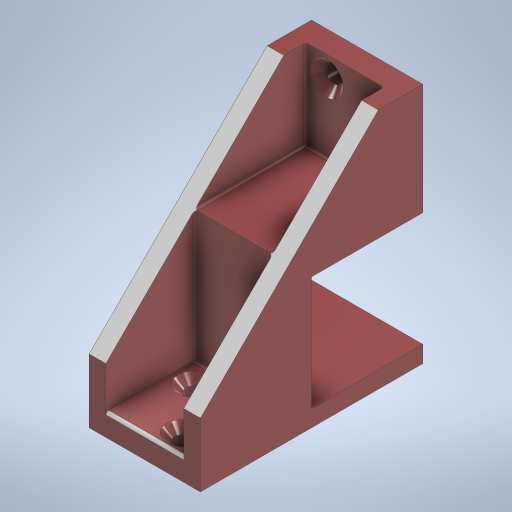
# Autodesk Inventor part: Uniont
Saved by Autodesk Inventor 2024 (Build 280153000, 153)
## iProperties
Created: 2023-07-08
Part Number: Uniont
Material: Genérico
Document SubType Name: Modeling
Designer: sergi
Density: 1 g/cm^3
Appearance: Valor por defecto
Author: sergi
Autodesk Inventor part; units mm, degrees
ref_plane "YZ Plane" through (0, 0, 0) normal (1, 0, 0) x (0, 1, 0)
ref_plane "XZ Plane" through (0, 0, 0) normal (0, 1, 0) x (-1, 0, 0)
ref_plane "Plano de trabajo1" through (0, 0, 0) normal (0, 0, 1) x (1, 0, 0)
sketch "Boceto1" plane through (0, 0, 0) normal (0, 0, 1) x (1, 0, 0)
  line L0 (-395, -200.5) -> (-395, -220.5) projected
  line L1 (-395, -220.5) -> (335, -220.5) projected
  line L2 (335, -200.5) -> (335, -220.5) projected
  line L3 (-395, -200.5) -> (335, -200.5) projected
  line L4 (-145, 767.5) -> (-145, -767.5) projected
  line L5 (-145, -767.5) -> (145, -767.5) projected
  line L6 (145, -767.5) -> (145, 767.5) projected
  line L7 (145, 767.5) -> (-145, 767.5) projected
  line L8 (335.5, -200) -> (335.5, -221)
  line L9 (335.5, -221) -> (-395.5, -221)
  line L10 (-395.5, -221) -> (-395.5, -200)
  line L11 (-395.5, -200) -> (335.5, -200)
  line L12 (-145, -200) -> (-145, -180)
  line L13 (-145, -180) -> (-125, -180)
  line L14 (-125, -180) -> (-125, -200)
  line L15 (-125, -200) -> (-145, -200)
  line L16 (-145, -200) -> (-145, -180)
  point P0 (0, 0)
  dimension "d0" = 0.5
  dimension "d1" = 20
  dimension "d2" = 20
  dimension "d3" = 20
  constraints: 18 end point, 3 point on line, 2 parallel, 1 horizontal, 1 perpendicular, 3 other
  measures "d0" distance between parallel lines of L3 L11
  measures "d1" distance of L12.start L12.end
  measures "d2" distance of L14.end L15.end
  measures "d3" distance of L13.end L14.end
extrude "Extrusión1" add sketch "Boceto1" along normal blind 4 contours L4 L13 L14 L11
sketch "Boceto3" plane through (0, 0, 4) normal (0, 0, 1) x (1, 0, 0)
  line L0 (-125, -180) -> (-145, -180) projected
  line L1 (-145, -180) -> (-145, -200) projected
  line L2 (-145, -200) -> (-125, -200) projected
  line L3 (-125, -200) -> (-125, -180) projected
  line L4 (-145, -200) -> (-125, -200)
  line L5 (-125, -200) -> (-125, -196)
  line L6 (-125, -196) -> (-145, -196)
  line L7 (-145, -196) -> (-145, -200)
  point P0 (0, 0)
  dimension "d6" = 4
  constraints: 8 end point, 2 parallel, 1 horizontal, 1 perpendicular, 1 point on line
  measures "d6" distance of L5.end L4.end
extrude "Extrusión2" add sketch "Boceto3" along normal blind 20 contours L3 L2 L1 L6
sketch "Boceto4" plane through (-145, -200, 0) normal (0, -1, 0) x (1, 0, 0)
  line L0 (0, 0) -> (20, 0) projected
  line L1 (20, 0) -> (20, 24) projected
  line L2 (0, 24) -> (20, 24) projected
  line L3 (0, 0) -> (0, 24) projected
  line L4 (0, 24) -> (20, 24) projected
  line L5 (20, 24) -> (0, 24)
  line L6 (0, 24) -> (0, 20)
  line L7 (0, 20) -> (20, 20)
  line L8 (20, 20) -> (20, 24)
  point P0 (145, 0)
  dimension "d9" = 4
  constraints: 8 end point, 2 parallel, 1 horizontal, 1 perpendicular, 1 point on line
  measures "d9" distance of L6.end L5.end
extrude "Extrusión3" add sketch "Boceto4" along normal blind 20.5 contours L3 L2 L1 L7
sketch "Boceto6" plane through (0, 0, 4) normal (0, 0, 1) x (1, 0, 0)
  line L0 (-145, -196) -> (-125, -196) projected
  line L1 (-125, -196) -> (-125, -180) projected
  line L2 (-125, -180) -> (-145, -180) projected
  line L3 (-145, -180) -> (-145, -196) projected
  line L4 (-145, -180) -> (-142, -180)
  line L5 (-142, -180) -> (-142, -196)
  line L6 (-142, -196) -> (-145, -196)
  line L7 (-145, -196) -> (-145, -180)
  line L8 (-125, -196) -> (-128, -196)
  line L9 (-128, -196) -> (-128, -180)
  line L10 (-128, -180) -> (-125, -180)
  line L11 (-125, -180) -> (-125, -196)
  point P0 (0, 0)
  dimension "d12" = 3
  dimension "d13" = 16
  dimension "d14" = 3
  constraints: 16 end point, 4 parallel, 2 horizontal, 2 perpendicular, 1 point on line
  measures "d12" distance of L5.end L6.end
  measures "d13" distance of L4.end L5.end
  measures "d14" distance of L9.end L10.end
extrude "Extrusión4" add sketch "Boceto6" along normal blind 20 contours L3 L2 L5 L0 | L9 L2 L1 L0
chamfer "Chaflán1" [suppressed]
sketch "Boceto7" plane through (0, 0, 4) normal (0, 0, 1) x (1, 0, 0)
  line L0 (-142, -180) -> (-142, -196) projected
  line L1 (-142, -196) -> (-128, -196) projected
  line L2 (-128, -196) -> (-128, -180) projected
  line L3 (-128, -180) -> (-142, -180) projected
  line L4 (-138.3, -192.3) -> (-138.3, -183.7)
  line L5 (-138.3, -183.7) -> (-131.7, -183.7)
  line L6 (-131.7, -183.7) -> (-131.7, -192.3)
  line L7 (-131.7, -192.3) -> (-138.3, -192.3)
  circle A0 centre (-138.3, -183.7) radius 3
  circle A1 centre (-131.7, -192.3) radius 3
  circle A2 centre (-138.3, -183.7) radius 1.65
  circle A3 centre (-131.7, -192.3) radius 1.65
  point P0 (0, 0)
  dimension "d20" = 3.7
  dimension "d21" = 6
  dimension "d22" = 6
  dimension "d23" = 3.3
  dimension "d24" = 3.3
  constraints: 8 end point, 4 centre point, 4 coincident, 3 other
  measures "d20" distance between parallel lines of L0 L4
  measures "d21" diameter of A0
  measures "d22" diameter of A1
  measures "d23" diameter of A2
  measures "d24" diameter of A3
hole "Agujero1" at (-138.3, -183.7, 4) at (-131.7, -192.3, 4) direction (0, 0, -1) diameter 3.2 end through all countersink diameter 6 countersink angle 90
sketch "Boceto8" plane through (-145, -220.5, 0) normal (0, -1, 0) x (1, 0, 0)
  line L0 (17, 24) -> (17, 4) projected
  line L1 (20, 20) -> (0, 20) projected
  line L2 (0, 0) -> (0, 20) projected
  line L3 (0, 0) -> (20, 0) projected
  line L4 (20, 0) -> (20, 20) projected
  line L5 (20, 20) -> (20, 24) projected
  line L6 (20, 24) -> (0, 24) projected
  line L7 (0, 24) -> (0, 20) projected
  line L8 (0, 20) -> (20, 20) projected
  point P0 (145, 0)
extrude "Extrusión5" add sketch "Boceto8" along normal blind 3
sketch "Boceto9" plane through (0, 0, 24) normal (0, 0, 1) x (1, 0, 0)
  line L0 (-145, -180) -> (-145, -223.5) projected
  line L1 (-125, -223.5) -> (-145, -223.5) projected
  line L2 (-125, -180) -> (-125, -223.5) projected
  line L3 (-128, -196) -> (-142, -196) projected
  line L4 (-145, -223.5) -> (-125, -223.5)
  line L5 (-125, -223.5) -> (-125, -219.5)
  line L6 (-125, -219.5) -> (-145, -219.5)
  line L7 (-145, -219.5) -> (-145, -223.5)
  line L8 (-125, -180) -> (-128, -180) projected
  line L9 (-128, -180) -> (-128, -196) projected
  line L10 (-142, -196) -> (-142, -180) projected
  line L11 (-142, -180) -> (-145, -180) projected
  point P0 (0, 0)
  dimension "d35" = 4
  constraints: 8 end point, 2 parallel, 1 horizontal, 1 perpendicular, 1 point on line
  measures "d35" distance of L5.end L4.end
extrude "Extrusión6" add sketch "Boceto9" along normal blind 16 contours L6 L2 L1 L0
sketch "Boceto10" plane through (-145, -219.5, 24) normal (0, 1, 0) x (1, 0, 0)
  line L0 (0, 0) -> (20, 0) projected
  line L1 (0, 0) -> (0, -16) projected
  line L2 (20, -16) -> (0, -16) projected
  line L3 (20, 0) -> (20, -16) projected
  line L4 (20, -16) -> (17, -16)
  line L5 (17, -16) -> (17, 0)
  line L6 (17, 0) -> (20, 0)
  line L7 (20, 0) -> (20, -16)
  line L8 (0, -16) -> (3, -16)
  line L9 (3, -16) -> (3, 0)
  line L10 (3, 0) -> (0, 0)
  line L11 (0, 0) -> (0, -16)
  point P0 (145, 24)
  point P1 (3, -16)
  point P2 (3, 0)
  point P3 (17, -16)
  dimension "d38" = 3
  dimension "d39" = 3
  dimension "d40" = 16
  constraints: 16 end point, 4 parallel, 2 horizontal, 2 perpendicular, 1 point on line
  measures "d38" distance of L5.end L6.end
  measures "d39" distance of L10.end L9.end
  measures "d40" distance of L9.end L8.end
extrude "Extrusión7" add sketch "Boceto10" along normal up to surface (39.5 mm away) contours L0 L9 L2 L1 | L0 L3 L2 L5
chamfer "Chaflán2" [suppressed]
chamfer "Chaflán3" [suppressed]
sketch "Boceto11" plane through (-142, -219.5, 24) normal (0, 1, 0) x (1, 0, 0)
  line L0 (0, 0) -> (0, -16) projected
  line L1 (14, -16) -> (0, -16) projected
  line L2 (14, -16) -> (14, 0) projected
  line L3 (0, 0) -> (14, 0) projected
  line L4 (3.7, -12.3) -> (3.7, -3.7)
  line L5 (3.7, -3.7) -> (10.3, -3.7)
  line L6 (10.3, -3.7) -> (10.3, -12.3)
  line L7 (10.3, -12.3) -> (3.7, -12.3)
  circle A0 centre (3.7, -3.7) radius 1.6
  circle A1 centre (10.3, -12.3) radius 1.6
  point P0 (142, 24)
  dimension "d49" = 3.7
  dimension "d50" = 3.2
  dimension "d51" = 3.2
  constraints: 8 end point, 2 centre point, 2 coincident, 3 other
  measures "d49" distance between parallel lines of L1 L7
  measures "d50" diameter of A0
  measures "d51" diameter of A1
hole "Agujero2" at (-131.7, -219.5, 36.3) at (-138.3, -219.5, 27.7) direction (0, -1, 0) diameter 3.2 end through all countersink diameter 6 countersink angle 90
fillet "Empalme2" radius 0.5 9 edges at (-135, -219.5, 40) (-142, -207.75, 24) (-128, -207.75, 24) (-135, -219.5, 24) (-142, -196, 14) (-135, -196, 4) (-142, -188, 4) (-128, -188, 4) (-128, -196, 14)
chamfer "Chaflán4" distance 32 angle 45 2 edges at (-143.5, -180, 40) (-126.5, -180, 40)
